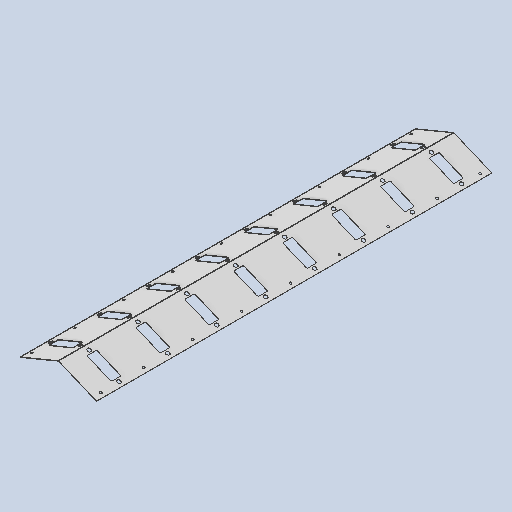
# Autodesk Inventor part: ДМФ 01 11 Барабан Лист крышка
Saved by Autodesk Inventor 2024.2 (Build 282272000, 272)
## iProperties
Created: 2024-04-28
Part Number: ДМФ 01 11 Барабан Лист крышка
Material: Generic
Document SubType Name: Sheet Metal
Designer: pokla
Density: 1 g/cm^3
Appearance: Default
Sheet Metal Rule: Default
Sheet Metal Width: 422,131 mm
Sheet Metal Length: 2020,000 mm
Sheet Metal Area: 852705,333 mm^2
Flat Pattern Width: 42.2131 cm
Flat Pattern Length: 202 cm
Flat Pattern Area: 8527.05 cm^2
Stock Number: Барабан_Лист_Крышка
Author: pokla
Autodesk Inventor part; units mm, degrees
ref_plane "YZ Plane" through (0, 0, 0) normal (1, 0, 0) x (0, 1, 0)
ref_plane "XZ Plane" through (0, 0, 0) normal (0, 1, 0) x (-1, 0, 0)
ref_plane "XY Plane" through (0, 0, 0) normal (0, 0, 1) x (1, 0, 0)
sketch "Sketch1" plane through (0, 0, 0) normal (0, 0, 1) x (1, 0, 0)
  line L0 (-196.316601, 196.316601) -> (0, 277.633599) construction
  line L1 (0, 277.633599) -> (196.316601, 196.316601) construction
  line L2 (196.316601, 196.316601) -> (277.633599, 0) construction
  line L3 (277.633599, 0) -> (196.316601, -196.316601) construction
  line L4 (196.316601, -196.316601) -> (0, -277.633599) construction
  line L5 (0, -277.633599) -> (-196.316601, -196.316601) construction
  line L6 (-196.316601, -196.316601) -> (-277.633599, 0) construction
  line L7 (-277.633599, 0) -> (-196.316601, 196.316601) construction
  line L8 (1.530734, 276.999549) -> (195.485109, 196.661016)
  line L9 (-1.530734, 276.999549) -> (-195.485109, 196.661016)
  arc A0 (1.530734, 276.999549) -> (-1.530734, 276.999549) centre (0, 273.304031) ccw
  point P0 (0, 0)
  point P1 (0, 0)
  dimension "d46" = 513
  dimension "d47" = 0.9
  dimension "d48" = 4
  measures "d46" distance between parallel lines of L7 L3
  measures "d47" distance of L0.start L9.end
  measures "d48" radius of A0
contour flange "Contour Flange2" sketch "Sketch1" thickness 2 bend radius 2 width 2020 along (0, 0, -1) mid plane no both sides no wall seen from (98.507921, 236.830282, 0) lies toward (-0.3826834, -0.9238795, 0) curves L8 A0 L9
bend "Bend4"
corner "Corner4"
sketch "Sketch12" plane through (1.530734, 276.999549, 0) normal (0.3826834, 0.9238795, 0) x (0.9238795, -0.3826834, 0)
  circle A0 centre (189.129, 40.75) radius 5.5
  line L0 (0, 0) -> (0, 2020)
  line L1 (209.934703, 0) -> (0, 0)
  circle A1 centre (189.129, 1979.25) radius 5.5
  line L2 (209.934703, 2020) -> (0, 2020)
  point P0 (104.588924, 0)
  dimension "d115" = 11
  dimension "d116" = 189.129
  dimension "d117" = 40.75
  dimension "d118" = 11
  dimension "d119" = 189.129
  dimension "d120" = 40.75
  constraints: 2 centre point
  measures "d115" diameter of A0
  measures "d116" distance from line of L0 A0.centre
  measures "d117" distance from line of L1 A0.centre
  measures "d118" diameter of A1
  measures "d119" distance from line of L0 A1.centre
  measures "d120" distance from line of L2 A1.centre
extrude "Extrusion5" cut sketch "Sketch12" against normal up to surface (2 mm away)
sketch "Sketch14" plane through (1.530734, 276.999549, 0) normal (0.3826834, 0.9238795, 0) x (0.9238795, -0.3826834, 0)
  line L0 (37.089, 1110) -> (172.089, 1110)
  line L1 (172.089, 1110) -> (172.089, 1160)
  line L2 (172.089, 1160) -> (37.089, 1160)
  line L3 (37.089, 1160) -> (37.089, 1110)
  line L4 (104.589, 1110) -> (104.589, 1160) construction
  line L5 (0, 0) -> (0, 2020) construction
  line L6 (22.089, 1135) -> (187.089, 1135) construction
  line L7 (13.689, 1139.849742) -> (22.089, 1144.699485)
  line L8 (22.089, 1144.699485) -> (30.489, 1139.849742)
  line L9 (30.489, 1139.849742) -> (30.489, 1130.150258)
  line L10 (30.489, 1130.150258) -> (22.089, 1125.300515)
  line L11 (22.089, 1125.300515) -> (13.689, 1130.150258)
  line L12 (13.689, 1130.150258) -> (13.689, 1139.849742)
  line L13 (178.689, 1139.849742) -> (187.089, 1144.699485)
  line L14 (187.089, 1144.699485) -> (195.489, 1139.849742)
  line L15 (195.489, 1139.849742) -> (195.489, 1130.150258)
  line L16 (195.489, 1130.150258) -> (187.089, 1125.300515)
  line L17 (187.089, 1125.300515) -> (178.689, 1130.150258)
  line L18 (178.689, 1130.150258) -> (178.689, 1139.849742)
  point P0 (104.588924, 0)
  point P1 (37.089, 1135)
  point P2 (172.089, 1135)
  point P3 (0, 1010)
  point P4 (104.589, 1135)
  point P5 (178.689, 1135)
  dimension "d131" = 135
  dimension "d132" = 50
  dimension "d135" = 125
  dimension "d136" = 104.589
  dimension "d160" = 165
  dimension "d161" = 16.8
  dimension "d162" = 16.8
  constraints: 36 end point, 8 midpoint, 3 parallel, 2 coincident, 2 horizontal, 1 perpendicular, 1 point on line, 26 other
  measures "d131" distance of L1.end L2.end
  measures "d132" distance of L2.end L0.start
  measures "d135" vertical distance of point (0, 1010) point (37.089, 1135)
  measures "d136" distance from line of L5 L4.start
  measures "d160" distance of L6.start L6.end
  measures "d161" distance between parallel lines of L9 L12
  measures "d162" distance between parallel lines of L15 L18
extrude "Extrusion7" cut sketch "Sketch14" against normal up to surface (2 mm away)
fillet "Fillet2" radius 5 4 edges at (35.4138, 261.8823, -1160) (35.4138, 261.8823, -1110) (160.1376, 210.2201, -1110) (160.1376, 210.2201, -1160)
pattern_circular "Circular Pattern1" count 2 over 45 about axis through (0, 0, -10) along (0, 0, 1) of "Extrusion7", "Fillet2"
pattern_linear "Rectangular Pattern5" count 8 spacing 250 along (0, 0, 1) of "Extrusion7", "Fillet2", "Circular Pattern1" first direction both ways yes
sketch "Sketch15" plane through (1.530734, 276.999549, 0) normal (0.3826834, 0.9238795, 0) x (0.9238795, -0.3826834, 0)
  circle A0 centre (189.129, 1010) radius 5.5
  line L0 (0, 0) -> (0, 2020) projected
  point P0 (104.588924, 0)
  point P1 (0, 1010)
  dimension "d146" = 11
  dimension "d147" = 189.129
  constraints: 1 centre point, 1 horizontal alignment, 1 midpoint
  measures "d146" diameter of A0
  measures "d147" distance from line of L0 A0.centre
extrude "Extrusion8" cut sketch "Sketch15" against normal through all
pattern_linear "Rectangular Pattern6" count 7 spacing 250 along (0, 0, 1) of "Extrusion8" first direction both ways yes
mirror "Mirror5" about plane through (0, 0, 0) normal (1, 0, 0) of "Extrusion8", "Extrusion5", "Rectangular Pattern6"
chamfer "Corner Chamfer1" distance 2 angle 45 1 edges at (-195.1024, 195.7371, 0)
fillet "Corner Round1" radius 2 1 edges at (195.1024, 195.7371, 0)
equation "\"d135\" = Барабан_Отступ_окна_от_середины"
equation "\"d46\" = Барабан_габарит_по_кассетам"
equation "\"d47\" = Барабан_отступ_развертки"
equation "\"d48\" = BendRadius + Thickness"
equation "\"d118\" = d115"
equation "\"d119\" = d116"
equation "\"d120\" = d117"
equation "\"d131\" = Барабан_Длина_окна"
equation "\"d132\" = Барабан_Ширина_окна"
equation "\"d136\" = Барабан_Расст_утановки_окна"
equation "\"d49\" = Thickness"
equation "\"d50\" = BendReliefWidth"
equation "\"d51\" = BendReliefDepth"
equation "\"d52\" = MinimumRemnant"
equation "\"d53\" = TransitionRadius"
equation "\"d54\" = Барабан_длина_листа"
equation "\"d55\" = BendRadius"
equation "\"d57\" = CornerReliefSize"
equation "\"d58\" = GapSize"
equation "\"d59\" = JacobiRadiusSize"
equation "\"BendRadius\" = Thickness"
equation "\"BendReliefWidth\" = Thickness"
equation "\"BendReliefDepth\" = 0.5 * Thickness"
equation "\"CornerReliefSize\" = 4 * Thickness"
equation "\"MinimumRemnant\" = 2 * Thickness"
equation "\"TransitionRadius\" = BendRadius"
equation "\"JacobiRadiusSize\" = BendRadius"
equation "\"GapSize\" = Thickness"
equation "\"Барабан_габарит_по_кассетам\" = 513"
equation "\"Барабан_отступ_развертки\" = 0.9"
equation "\"Thickness\" = 2"
equation "\"Барабан_Длина_окна\" = 135"
equation "\"Барабан_Ширина_окна\" = 50"
equation "\"Барабан_Расст_утановки_окна\" = 104.589"
equation "\"Барабан_длина_листа\" = 2020"
equation "\"Барабан_Отступ_окна_от_середины\" = 125"
body "Solid2"
